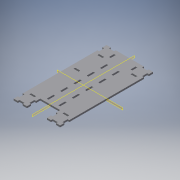
# Autodesk Inventor part: Part1
Saved by Autodesk Inventor 2018 (Build 220112000, 112)
## iProperties
Created: 2018-05-14
Part Number: Part1
Material: Generic
Document SubType Name: Modeling
Designer: Administrator
Density: 1 g/cm^3
Appearance: Default
Author: Administrator
Autodesk Inventor part; units mm, degrees
ref_plane "YZ Plane" through (0, 0, 0) normal (1, 0, 0) x (0, 1, 0)
ref_plane "XZ Plane" through (0, 0, 0) normal (0, 1, 0) x (-1, 0, 0)
ref_plane "XY Plane" through (0, 0, 0) normal (0, 0, 1) x (1, 0, 0)
sketch "Sketch1" plane through (0, 0, 0) normal (0, 1, 0) x (-1, 0, 0)
  line L0 (-5.1509, 7.7422) -> (-94.0509, 7.7422)
  line L1 (-94.0509, 7.7422) -> (-94.0509, -170.0578)
  line L2 (-94.0509, -170.0578) -> (-5.1509, -170.0578)
  line L3 (-5.1509, -170.0578) -> (-5.1509, 7.7422)
  point P0 (0, 0)
  dimension "d0" = 177.8
  dimension "d1" = 88.9
  constraints: 8 end point, 2 parallel, 1 horizontal, 1 perpendicular
  measures "d0" distance between parallel lines of L2 L0
  measures "d1" distance between parallel lines of L1 L3
extrude "Extrusion1" add sketch "Sketch1" along normal blind 3.175
sketch "Sketch2" plane through (0, 3.175, 0) normal (0, 1, 0) x (1, 0, 0)
  line L0 (5.1509, -7.7422) -> (94.0509, -7.7422) projected
  line L1 (13.0884, -7.7422) -> (22.6134, -7.7422)
  line L2 (22.6134, -7.7422) -> (22.6134, -4.5672)
  line L3 (22.6134, -4.5672) -> (13.0884, -4.5672)
  line L4 (13.0884, -4.5672) -> (13.0884, -7.7422)
  line L5 (5.1509, 170.0578) -> (5.1509, -7.7422) projected
  line L6 (5.1509, 0.1953) -> (8.3259, 0.1953)
  line L7 (8.3259, 0.1953) -> (8.3259, 9.7203)
  line L8 (8.3259, 9.7203) -> (5.1509, 9.7203)
  line L9 (5.1509, 9.7203) -> (5.1509, 0.1953)
  line L10 (13.0884, 14.4828) -> (22.6134, 14.4828)
  line L11 (22.6134, 14.4828) -> (22.6134, 17.6578)
  line L12 (22.6134, 17.6578) -> (13.0884, 17.6578)
  line L13 (13.0884, 17.6578) -> (13.0884, 14.4828)
  line L14 (27.3759, 0.1953) -> (30.5509, 0.1953)
  line L15 (30.5509, 0.1953) -> (30.5509, 9.7203)
  line L16 (30.5509, 9.7203) -> (27.3759, 9.7203)
  line L17 (27.3759, 9.7203) -> (27.3759, 0.1953)
  line L18 (94.0509, -7.7422) -> (94.0509, 170.0578) projected
  line L19 (94.0509, 0.1953) -> (90.8759, 0.1953)
  line L20 (90.8759, 0.1953) -> (90.8759, 9.7203)
  line L21 (90.8759, 9.7203) -> (94.0509, 9.7203)
  line L22 (94.0509, 9.7203) -> (94.0509, 0.1953)
  line L23 (86.1134, -4.5672) -> (76.5884, -4.5672)
  line L24 (76.5884, -4.5672) -> (76.5884, -7.7422)
  line L25 (76.5884, -7.7422) -> (86.1134, -7.7422)
  line L26 (86.1134, -7.7422) -> (86.1134, -4.5672)
  line L27 (71.8259, 0.1953) -> (68.6509, 0.1953)
  line L28 (68.6509, 0.1953) -> (68.6509, 9.7203)
  line L29 (68.6509, 9.7203) -> (71.8259, 9.7203)
  line L30 (71.8259, 9.7203) -> (71.8259, 0.1953)
  line L31 (86.1134, 14.4828) -> (76.5884, 14.4828)
  line L32 (76.5884, 14.4828) -> (76.5884, 17.6578)
  line L33 (76.5884, 17.6578) -> (86.1134, 17.6578)
  line L34 (86.1134, 17.6578) -> (86.1134, 14.4828)
  point P0 (0, 0)
  dimension "d4" = 7.9375
  dimension "d5" = 3.175
  dimension "d6" = 9.525
  dimension "d7" = 7.9375
  dimension "d8" = 3.175
  dimension "d9" = 9.525
  dimension "d10" = 3.175
  dimension "d11" = 7.9375
  dimension "d12" = 3.175
  dimension "d13" = 7.9375
  dimension "d14" = 3.175
  dimension "d15" = 7.9375
  dimension "d16" = 9.525
  dimension "d17" = 7.9375
  dimension "d18" = 3.175
  dimension "d21" = 3.175
  dimension "d22" = 3.175
  dimension "d23" = 7.9375
  dimension "d30" = 9.525
  dimension "d33" = 7.9375
  dimension "d34" = 7.9375
  dimension "d35" = 9.525
  constraints: 64 end point, 16 parallel, 8 horizontal, 8 perpendicular, 4 point on line
  measures "d4" distance between parallel lines of L5 L4
  measures "d5" distance between parallel lines of L0 L3
  measures "d6" distance between parallel lines of L4 L2
  measures "d7" distance between parallel lines of L0 L6
  measures "d8" distance between parallel lines of L5 L7
  measures "d9" distance between parallel lines of L8 L6
  measures "d10" distance between parallel lines of L10 L12
  measures "d11" distance between parallel lines of L12 L8
  measures "d12" distance between parallel lines of L15 L17
  measures "d13" distance between parallel lines of L15 L2
  measures "d14" distance between parallel lines of L22 L20
  measures "d15" distance between parallel lines of L18 L26
  measures "d16" distance from line of L24.end L26
  measures "d17" distance between parallel lines of L24 L28
  measures "d18" distance between parallel lines of L28 L30
  measures "d21" distance between parallel lines of L33 L31
  measures "d22" distance between parallel lines of L25 L23
  measures "d23" distance between parallel lines of L33 L29
  measures "d30" distance between parallel lines of L14 L16
  measures "d33" distance from line of L11.end L16
  measures "d34" distance between parallel lines of L21 L33
  measures "d35" distance between parallel lines of L21 L19
extrude "Extrusion2" cut sketch "Sketch2" against normal blind 3.175
ref_plane "Work Plane1" through (22.6134, 0, -81.1578) normal (0, 0, 1) x (1, 0, 0)
sketch "Sketch3" plane through (0, 3.175, 0) normal (0, 1, 0) x (1, 0, 0)
  line L0 (22.6134, -7.7422) -> (76.5884, -7.7422) projected
  line L1 (30.5509, -7.7422) -> (68.6509, -7.7422)
  line L2 (68.6509, -7.7422) -> (68.6509, 17.6578)
  line L3 (68.6509, 17.6578) -> (30.5509, 17.6578)
  line L4 (30.5509, 17.6578) -> (30.5509, -7.7422)
  line L5 (5.1509, 170.0578) -> (5.1509, 9.7203) projected
  line L6 (94.0509, -7.7422) -> (94.0509, 170.0578) projected
  point P0 (0, 0)
  point P1 (94.0509, 9.7203)
  dimension "d26" = 25.4
  dimension "d27" = 25.4
  dimension "d28" = 25.4
  constraints: 8 end point, 2 parallel, 1 horizontal, 1 perpendicular, 1 point on line
  measures "d26" distance between parallel lines of L0 L3
  measures "d27" distance between parallel lines of L5 L4
  measures "d28" distance between parallel lines of L6 L2
extrude "Extrusion3" cut sketch "Sketch3" against normal blind 3.175
mirror "Mirror3" about plane through (22.6134, 0, -81.1578) normal (0, 0, 1) of "Extrusion2"
ref_plane "Work Plane3" through (49.6009, 0, -9.7203) normal (1, 0, 0) x (0, 0, -1)
sketch "Sketch5" plane through (0, 3.175, 0) normal (0, 1, 0) x (1, 0, 0)
  line L0 (36.9009, 49.4078) -> (40.0759, 49.4078)
  line L1 (40.0759, 49.4078) -> (40.0759, 62.1078)
  line L2 (40.0759, 62.1078) -> (36.9009, 62.1078)
  line L3 (36.9009, 62.1078) -> (36.9009, 49.4078)
  line L4 (49.6009, 205.6178) -> (49.6009, -43.3022) projected
  line L5 (36.9009, 36.7078) -> (40.0759, 36.7078)
  line L6 (40.0759, 36.7078) -> (40.0759, 24.0078)
  line L7 (40.0759, 24.0078) -> (36.9009, 24.0078)
  line L8 (36.9009, 24.0078) -> (36.9009, 36.7078)
  line L9 (30.5509, 17.6578) -> (68.6509, 17.6578) projected
  line L10 (36.9009, 74.8078) -> (40.0759, 74.8078)
  line L11 (40.0759, 74.8078) -> (40.0759, 87.5078)
  line L12 (40.0759, 87.5078) -> (36.9009, 87.5078)
  line L13 (36.9009, 87.5078) -> (36.9009, 74.8078)
  line L14 (36.9009, 100.2078) -> (40.0759, 100.2078)
  line L15 (40.0759, 100.2078) -> (40.0759, 112.9078)
  line L16 (40.0759, 112.9078) -> (36.9009, 112.9078)
  line L17 (36.9009, 112.9078) -> (36.9009, 100.2078)
  line L18 (36.9009, 125.6078) -> (40.0759, 125.6078)
  line L19 (40.0759, 125.6078) -> (40.0759, 138.3078)
  line L20 (40.0759, 138.3078) -> (36.9009, 138.3078)
  line L21 (36.9009, 138.3078) -> (36.9009, 125.6078)
  point P0 (0, 0)
  dimension "d36" = 9.525
  dimension "d37" = 3.175
  dimension "d38" = 12.7
  dimension "d39" = 12.7
  dimension "d40" = 12.7
  dimension "d41" = 6.35
  dimension "d42" = 12.7
  dimension "d43" = 12.7
  dimension "d44" = 12.7
  dimension "d45" = 12.7
  dimension "d46" = 12.7
  dimension "d47" = 12.7
  constraints: 40 end point, 10 parallel, 5 horizontal, 5 perpendicular, 4 point on line
  measures "d36" distance between parallel lines of L1 L4
  measures "d37" distance between parallel lines of L1 L3
  measures "d38" distance between parallel lines of L2 L0
  measures "d39" distance between parallel lines of L0 L5
  measures "d40" distance between parallel lines of L5 L7
  measures "d41" distance between parallel lines of L9 L7
  measures "d42" distance between parallel lines of L2 L10
  measures "d43" distance between parallel lines of L10 L12
  measures "d44" distance between parallel lines of L12 L14
  measures "d45" distance between parallel lines of L14 L16
  measures "d46" distance between parallel lines of L16 L18
  measures "d47" distance between parallel lines of L18 L20
extrude "Extrusion4" cut sketch "Sketch5" against normal blind 3.175
mirror "Mirror4" about plane through (49.6009, 0, -9.7203) normal (1, 0, 0) of "Extrusion4"
sketch "Sketch6" plane through (0, 3.175, 0) normal (0, 1, 0) x (1, 0, 0)
  line L0 (22.6134, 102.3414) -> (13.0884, 102.3414)
  line L1 (13.0884, 102.3414) -> (13.0884, 99.1664)
  line L2 (13.0884, 99.1664) -> (22.6134, 99.1664)
  line L3 (22.6134, 99.1664) -> (22.6134, 102.3414)
  line L4 (22.6134, 144.6578) -> (13.0884, 144.6578) projected
  line L5 (22.6134, 147.8328) -> (22.6134, 144.6578) projected
  line L6 (13.0884, 144.6578) -> (13.0884, 147.8328) projected
  point P0 (0, 0)
  dimension "d50" = 3.175
  dimension "d51" = 42.3164
  constraints: 8 end point, 2 collinear, 2 parallel, 1 horizontal, 1 perpendicular
  measures "d50" distance between parallel lines of L2 L0
  measures "d51" distance between parallel lines of L0 L4
extrude "Extrusion5" cut sketch "Sketch6" against normal blind 3.175
sketch "Sketch7" plane through (0, 3.175, 0) normal (0, 1, 0) x (1, 0, 0)
  line L0 (13.0884, 17.6578) -> (22.6134, 17.6578) projected
  line L1 (22.6134, 17.6578) -> (13.0884, 17.6578)
  line L2 (13.0884, 17.6578) -> (13.0884, 20.8328)
  line L3 (13.0884, 20.8328) -> (22.6134, 20.8328)
  line L4 (22.6134, 20.8328) -> (22.6134, 17.6578)
  line L5 (5.1509, 152.5953) -> (5.1509, 9.7203) projected
  line L6 (5.1509, 25.5953) -> (8.3259, 25.5953)
  line L7 (8.3259, 25.5953) -> (8.3259, 35.1203)
  line L8 (8.3259, 35.1203) -> (5.1509, 35.1203)
  line L9 (5.1509, 35.1203) -> (5.1509, 25.5953)
  line L10 (30.5509, 25.5953) -> (27.3759, 25.5953)
  line L11 (27.3759, 25.5953) -> (27.3759, 35.1203)
  line L12 (27.3759, 35.1203) -> (30.5509, 35.1203)
  line L13 (30.5509, 35.1203) -> (30.5509, 25.5953)
  line L14 (13.0884, 39.8828) -> (22.6134, 39.8828)
  line L15 (22.6134, 39.8828) -> (22.6134, 43.0578)
  line L16 (22.6134, 43.0578) -> (13.0884, 43.0578)
  line L17 (13.0884, 43.0578) -> (13.0884, 39.8828)
  point P0 (0, 0)
  dimension "d54" = 3.175
  dimension "d55" = 3.175
  dimension "d56" = 7.9375
  dimension "d57" = 9.525
  dimension "d58" = 3.175
  dimension "d59" = 25.4
  dimension "d60" = 3.175
  dimension "d61" = 25.4
  constraints: 32 end point, 8 parallel, 4 horizontal, 4 perpendicular, 1 point on line
  measures "d54" distance between parallel lines of L0 L3
  measures "d55" distance between parallel lines of L5 L7
  measures "d56" distance between parallel lines of L0 L6
  measures "d57" distance between parallel lines of L6 L8
  measures "d58" distance between parallel lines of L11 L13
  measures "d59" distance between parallel lines of L9 L13
  measures "d60" distance between parallel lines of L14 L16
  measures "d61" distance between parallel lines of L0 L16
extrude "Extrusion6" cut sketch "Sketch7" against normal blind 3.175
mirror "Mirror5" about plane through (49.6009, 0, -9.7203) normal (1, 0, 0) of "Extrusion6"
mirror "Mirror6" about plane through (22.6134, 0, -81.1578) normal (0, 0, 1) of "Extrusion6", "Mirror5"
sketch "Sketch8" plane through (0, 3.175, 0) normal (0, 1, 0) x (1, 0, 0)
  line L0 (13.0884, 43.0578) -> (13.0884, 39.8828) projected
  line L1 (13.0884, 43.0578) -> (22.6134, 43.0578)
  line L2 (22.6134, 43.0578) -> (22.6134, 46.2328)
  line L3 (22.6134, 46.2328) -> (13.0884, 46.2328)
  line L4 (13.0884, 46.2328) -> (13.0884, 43.0578)
  line L5 (27.3759, 50.9953) -> (30.5509, 50.9953)
  line L6 (30.5509, 50.9953) -> (30.5509, 60.5203)
  line L7 (30.5509, 60.5203) -> (27.3759, 60.5203)
  line L8 (27.3759, 60.5203) -> (27.3759, 50.9953)
  line L9 (5.1509, 127.1953) -> (5.1509, 35.1203) projected
  line L10 (5.1509, 127.1953) -> (5.1509, 35.1203) projected
  line L11 (8.3259, 60.5203) -> (5.1509, 60.5203)
  line L12 (5.1509, 60.5203) -> (5.1509, 50.9953)
  line L13 (5.1509, 50.9953) -> (8.3259, 50.9953)
  line L14 (8.3259, 50.9953) -> (8.3259, 60.5203)
  line L15 (13.0884, 65.2828) -> (22.6134, 65.2828)
  line L16 (22.6134, 65.2828) -> (22.6134, 68.4578)
  line L17 (22.6134, 68.4578) -> (13.0884, 68.4578)
  line L18 (13.0884, 68.4578) -> (13.0884, 65.2828)
  point P0 (0, 0)
  dimension "d64" = 3.175
  dimension "d65" = 3.175
  dimension "d66" = 9.525
  dimension "d67" = 7.9375
  dimension "d68" = 25.4
  dimension "d69" = 3.175
  dimension "d70" = 25.4
  constraints: 32 end point, 8 parallel, 4 horizontal, 4 perpendicular, 1 point on line
  measures "d64" distance between parallel lines of L1 L3
  measures "d65" distance between parallel lines of L6 L8
  measures "d66" distance between parallel lines of L5 L7
  measures "d67" distance between parallel lines of L1 L5
  measures "d68" distance between parallel lines of L9 L6
  measures "d69" distance between parallel lines of L15 L17
  measures "d70" distance between parallel lines of L1 L17
extrude "Extrusion7" cut sketch "Sketch8" against normal blind 3.175
mirror "Mirror7" about plane through (49.6009, 0, -9.7203) normal (1, 0, 0) of "Extrusion7"
body "Solid1"
